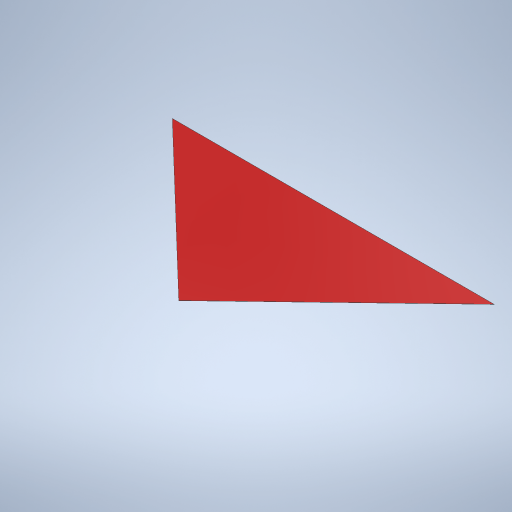
# Autodesk Inventor part: keepout - top B
Saved by Autodesk Inventor 2023 (Build 270158000, 158)
## iProperties
Created: 2023-03-02
Part Number: keepout - top B
Material: Generic
Document SubType Name: Modeling
Designer: Caleb
Density: 1 g/cm^3
Appearance: Default
Author: Caleb
Autodesk Inventor part; units mm, degrees
ref_plane "YZ Plane" through (0, 0, 0) normal (1, 0, 0) x (0, 1, 0)
ref_plane "XZ Plane" through (0, 0, 0) normal (0, 1, 0) x (-1, 0, 0)
ref_plane "XY Plane" through (0, 0, 0) normal (0, 0, 1) x (1, 0, 0)
sketch "Sketch1" plane through (0, 0, 0) normal (0, 1, 0) x (-1, 0, 0)
  line L0 (12.5, 0) -> (-12.5, 0)
  line L1 (-12.5, 0) -> (0, 12)
  line L2 (0, 12) -> (12.5, 0)
  point P0 (0, 0)
  dimension "d0" = 25
  dimension "d1" = 12
  dimension "d2" = 12.5
  constraints: 6 end point, 1 horizontal, 1 midpoint, 1 vertical alignment
  measures "d0" distance of L0.start L0.end
  measures "d1" distance from line of L1.end L0
  measures "d2" horizontal distance of L0.start L1.end
extrude "Extrusion1" add sketch "Sketch1" along normal blind 0.01
equation "\"d2\" = 0.5 * d0"
body "Solid1"
